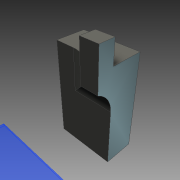
# Autodesk Inventor part: Rangelink Reciever
Saved by Autodesk Inventor 2013 SP1 (Build 170176100, 176)
## iProperties
Created: 2013-03-10
Part Number: Rangelink Reciever
Material: Generic
Document SubType Name: Modeling
Designer: fixer
Density: 0.707036 g/cm^3
Mass: 17.3 g
Surface Area: 59.8196 cm^2
Volume: 24.4684 cm^3
Author: fixer
Autodesk Inventor part; units mm, degrees
ref_plane "YZ Plane" through (0, 0, 0) normal (1, 0, 0) x (0, 1, 0)
ref_plane "XZ Plane" through (0, 0, 0) normal (0, 1, 0) x (-1, 0, 0)
ref_plane "XY Plane" through (0, 0, 0) normal (0, 0, 1) x (1, 0, 0)
sketch "Sketch1" plane through (0, 0, 0) normal (0, 0, 1) x (1, 0, 0)
  line L0 (52.1911, 179.7031) -> (21.9651, 179.7031)
  line L1 (21.9651, 179.7031) -> (21.9651, 130.4271)
  line L2 (21.9651, 130.4271) -> (52.1911, 130.4271)
  line L3 (52.1911, 130.4271) -> (52.1911, 179.7031)
  point P0 (0, 0)
  dimension "d0" = 30.226
  dimension "d1" = 49.276
  constraints: 8 end point, 2 parallel, 1 horizontal, 1 perpendicular
  measures "d0" distance of L0.start L0.end
  measures "d1" distance of L0.end L1.end
extrude "Extrusion1" add sketch "Sketch1" along normal blind 15.24
sketch "Sketch2" plane through (0, 0, 15.24) normal (0, 0, 1) x (1, 0, 0)
  line L0 (52.1911, 179.7031) -> (52.1911, 130.4271) projected
  line L1 (21.9651, 179.7031) -> (52.1911, 179.7031) projected
  line L2 (52.1911, 171.0671) -> (43.5551, 171.0671)
  line L3 (43.5551, 171.0671) -> (43.5551, 190.3711)
  line L4 (43.5551, 190.3711) -> (52.1911, 190.3711)
  line L5 (52.1911, 190.3711) -> (52.1911, 171.0671)
  point P0 (0, 0)
  dimension "d4" = 8.636
  dimension "d5" = 8.636
  dimension "d6" = 10.668
  constraints: 8 end point, 2 parallel, 1 horizontal, 1 perpendicular, 1 point on line
  measures "d4" distance of L2.start L2.end
  measures "d5" distance between parallel lines of L1 L2
  measures "d6" distance between parallel lines of L1 L4
extrude "Extrusion2" add sketch "Sketch2" along normal blind 7.366
fillet "Fillet1" radius 12.7 2 edges at (43.5551, 175.3851, 15.24) (47.8731, 171.0671, 15.24)
body "Solid1"
